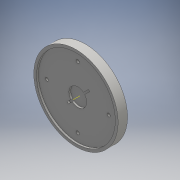
# Autodesk Inventor part: Motor Mount Fancy
Saved by Autodesk Inventor 2016 SP1 (Build 200210100, 210)
## iProperties
Created: 2017-05-01
Part Number: Motor Mount Fancy
Material: Generic
Document SubType Name: Modeling
Designer: mundhend06
Density: 1 g/cm^3
Appearance: Default
Author: mundhend06
Autodesk Inventor part; units mm, degrees
ref_plane "YZ Plane" through (0, 0, 0) normal (1, 0, 0) x (0, 1, 0)
ref_plane "XZ Plane" through (0, 0, 0) normal (0, 1, 0) x (-1, 0, 0)
ref_plane "XY Plane" through (0, 0, 0) normal (0, 0, 1) x (1, 0, 0)
sketch "Sketch1" plane through (0, 0, 0) normal (0, 1, 0) x (-1, 0, 0)
  circle A0 centre (0, 0) radius 22.5
  dimension "d0" = 45
  constraints: 1 centre point, 1 coincident
  measures "d0" diameter of A0
extrude "Extrusion1" add sketch "Sketch1" along normal blind 5
sketch "Sketch2" plane through (0, 5, 0) normal (0, 1, 0) x (1, 0, 0)
  line L0 (0, 0) -> (0, 8) construction
  line L1 (0, 0) -> (0, -8) construction
  circle A0 centre (0, 8) radius 1.9
  circle A1 centre (0, 0) radius 1.9
  circle A2 centre (0, -8) radius 1.9
  dimension "d3" = 8
  dimension "d4" = 8
  dimension "d5" = 3.8
  dimension "d6" = 3.8
  dimension "d7" = 3.8
  constraints: 4 end point, 3 centre point, 3 coincident, 2 vertical
  measures "d3" distance of L0.start L0.end
  measures "d4" distance of L0.start L1.end
  measures "d5" diameter of A0
  measures "d6" diameter of A1
  measures "d7" diameter of A2
extrude "Extrusion2" add sketch "Sketch2" along normal blind 10
sketch "Sketch7" plane through (0, 0, 0) normal (0, -1, 0) x (1, 0, 0)
  circle A0 centre (0, 0) radius 16.5 construction
  circle A1 centre (0, 16.5) radius 0.85
  circle A2 centre (16.5, 0) radius 0.85
  circle A3 centre (-16.5, 0) radius 0.85
  circle A4 centre (0, -16.5) radius 0.85
  dimension "d42" = 33
  dimension "d43" = 1.7
  dimension "d44" = 1.7
  dimension "d45" = 1.7
  dimension "d46" = 1.7
  constraints: 5 centre point, 4 point on circle, 1 coincident
  measures "d42" diameter of A0
  measures "d43" diameter of A1
  measures "d44" diameter of A2
  measures "d45" diameter of A3
  measures "d46" diameter of A4
extrude "Extrusion6" cut sketch "Sketch7" against normal blind 5
sketch "Sketch8" plane through (0, 0, 0) normal (0, -1, 0) x (1, 0, 0)
  circle A0 centre (0, 0) radius 21
  dimension "d49" = 42
  constraints: 1 centre point, 1 coincident
  measures "d49" diameter of A0
extrude "Extrusion7" cut sketch "Sketch8" against normal blind 1
sketch "Sketch9" plane through (0, 1, 0) normal (0, -1, 0) x (1, 0, 0)
  circle A0 centre (0, 0) radius 4.75
  line L0 (0, 0) -> (6, 0) construction
  line L1 (6, 0) -> (6, 6) construction
  line L2 (6, 6) -> (0, 6) construction
  line L3 (0, 6) -> (0, 0) construction
  line L4 (0, 0) -> (6, 6) construction
  line L5 (6, 6) -> (5.6464, 6.3536) construction
  line L6 (5.6464, 6.3536) -> (-5.6673, -4.9602)
  line L7 (-5.6673, -4.9602) -> (-4.9602, -5.6673)
  line L8 (-4.9602, -5.6673) -> (6.3536, 5.6464)
  line L9 (6.3536, 5.6464) -> (5.6464, 6.3536)
  dimension "d52" = 9.5
  dimension "d53" = 6
  dimension "d54" = 6
  dimension "d55" = 0.5
  dimension "d56" = 16
  dimension "d57" = 1
  constraints: 20 end point, 3 perpendicular, 2 parallel, 1 centre point, 1 coincident, 1 collinear, 1 horizontal
  measures "d52" diameter of A0
  measures "d53" distance of L1.end L2.end
  measures "d54" distance of L0.end L1.end
  measures "d55" distance of L1.end L5.end
  measures "d56" distance of L5.end L6.end
  measures "d57" distance of L6.end L7.end
extrude "Extrusion8" cut sketch "Sketch9" against normal blind 1
body "Solid1"
